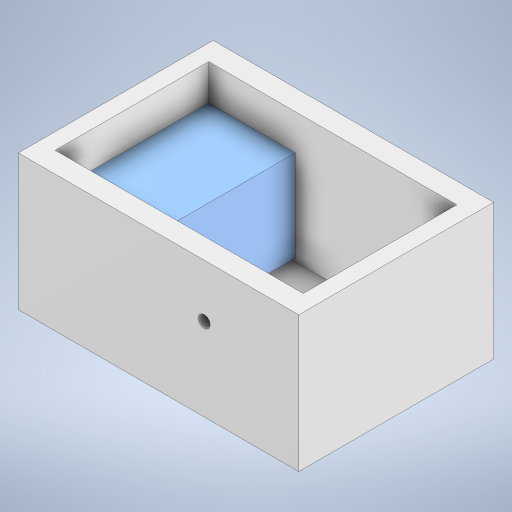
# Autodesk Inventor part: JunctionBox
Saved by Autodesk Inventor 2024.2 (Build 282272000, 272)
## iProperties
Created: 2024-01-15
Part Number: JunctionBox
Material: ABS Plastic
Document SubType Name: Modeling
Designer: airso
Density: 1.06 g/cm^3
Appearance: Smooth - White
Author: airso
Autodesk Inventor part; units mm, degrees
ref_plane "YZ Plane" through (0, 0, 0) normal (1, 0, 0) x (0, 1, 0)
ref_plane "XZ Plane" through (0, 0, 0) normal (0, 1, 0) x (-1, 0, 0)
ref_plane "XY Plane" through (0, 0, 0) normal (0, 0, 1) x (1, 0, 0)
sketch "Sketch1" plane through (0, 0, 0) normal (0, 1, 0) x (-1, 0, 0)
  line L0 (133.35, 82.55) -> (-133.35, 82.55)
  line L1 (-133.35, 82.55) -> (-133.35, -82.55)
  line L2 (-133.35, -82.55) -> (133.35, -82.55)
  line L3 (133.35, -82.55) -> (133.35, 82.55)
  line L4 (133.35, 82.55) -> (-133.35, -82.55) construction
  line L5 (-133.35, 82.55) -> (133.35, -82.55) construction
  line L6 (-150.8125, 104.775) -> (150.8125, 104.775)
  line L7 (150.8125, 104.775) -> (150.8125, -104.775)
  line L8 (150.8125, -104.775) -> (-150.8125, -104.775)
  line L9 (-150.8125, -104.775) -> (-150.8125, 104.775)
  line L10 (-150.8125, 104.775) -> (150.8125, -104.775) construction
  line L11 (150.8125, 104.775) -> (-150.8125, -104.775) construction
  point P0 (0, 0)
  dimension "d0" = 165.1
  dimension "d1" = 266.7
  dimension "d2" = 209.55
  dimension "d3" = 301.625
  constraints: 24 end point, 4 midpoint, 4 parallel, 2 horizontal, 2 perpendicular
  measures "d0" distance of L2.end L0.start
  measures "d1" distance of L1.end L2.end
  measures "d2" distance of L6.end L7.end
  measures "d3" distance of L6.start L6.end
extrude "Extrusion1" add sketch "Sketch1" along normal blind 146.05
sketch "Sketch2" plane through (0, 0, 0) normal (0, -1, 0) x (1, 0, 0)
  line L0 (133.35, 82.55) -> (-133.35, 82.55) projected
  line L1 (-133.35, -82.55) -> (133.35, -82.55) projected
  line L2 (-133.35, 82.55) -> (133.35, 82.55)
  line L3 (133.35, 82.55) -> (133.35, -82.55)
  line L4 (133.35, -82.55) -> (-133.35, -82.55)
  line L5 (-133.35, -82.55) -> (-133.35, 82.55)
  point P0 (0, 0)
  point P1 (133.35, 82.55)
  point P2 (-133.35, -82.55)
  constraints: 8 end point, 2 parallel, 1 horizontal, 1 perpendicular
extrude "Extrusion2" add sketch "Sketch2" against normal blind 3.175
sketch "Sketch3" plane through (0, 3.175, 0) normal (0, 1, 0) x (1, 0, 0)
  line L0 (-133.35, -82.55) -> (-133.35, 82.55) projected
  line L1 (-133.35, 82.55) -> (133.35, 82.55) projected
  line L2 (-133.35, -82.55) -> (133.35, -82.55)
  line L3 (133.35, -82.55) -> (133.35, 82.55)
  line L4 (133.35, 82.55) -> (-133.35, 82.55)
  line L5 (-133.35, 82.55) -> (-133.35, -82.55)
  line L6 (130.175, -79.375) -> (-130.175, -79.375)
  line L7 (-130.175, -79.375) -> (-130.175, 79.375)
  line L8 (-130.175, 79.375) -> (130.175, 79.375)
  line L9 (130.175, 79.375) -> (130.175, -79.375)
  point P0 (0, 0)
  dimension "d8" = 3.175
  constraints: 16 end point, 4 parallel, 2 perpendicular, 1 horizontal, 3 other
  measures "d8" distance between parallel lines of L2 L6
extrude "Extrusion3" add sketch "Sketch3" along normal blind 6.35 contours L6 L7 L8 L9
sketch "Sketch5" plane through (-133.35, 146.05, 82.55) normal (1, 0, 0) x (0, 0, -1)
  line L0 (0, -38.481) -> (165.1, -38.481)
  line L1 (165.1, -38.481) -> (14.224, -38.481)
  line L2 (14.224, -38.481) -> (14.224, -136.525)
  line L3 (14.224, -136.525) -> (165.1, -136.525)
  line L4 (165.1, -136.525) -> (165.1, -38.481)
  point P0 (82.55, -146.05)
  point P1 (165.1, -142.875)
  dimension "d15" = 98.044
  dimension "d16" = 150.876
  dimension "d19" = 6.35
  constraints: 10 end point, 2 parallel, 1 horizontal, 1 perpendicular
  measures "d15" distance of L1.end L2.end
  measures "d16" distance of L2.end L3.end
  measures "d19" distance from line of point (165.1, -142.875) L3
extrude "Extrusion5" add sketch "Sketch5" along normal blind 92.964
sketch "Sketch6" plane through (0, 9.525, 0) normal (0, 1, 0) x (1, 0, 0)
  line L0 (62.8142, 28.702) -> (-34.036, 28.702)
  line L1 (-34.036, 28.702) -> (-34.036, -79.375)
  line L2 (-34.036, -79.375) -> (62.8142, -79.375)
  line L3 (62.8142, -79.375) -> (62.8142, 28.702)
  line L4 (-130.175, -79.375) -> (130.175, -79.375) projected
  line L5 (-40.386, 82.55) -> (-40.386, -68.326) projected
  point P0 (0, 0)
  dimension "d20" = 108.077
  dimension "d21" = 96.8502
  dimension "d61" = 0
  dimension "d62" = 6.35
  constraints: 8 end point, 2 parallel, 1 horizontal, 1 perpendicular
  measures "d20" distance of L2.end L0.start
  measures "d21" distance of L1.end L2.end
  measures "d61" distance between parallel lines of L4 L2
  measures "d62" distance between parallel lines of L5 L1
extrude "Extrusion6" add sketch "Sketch6" along normal blind 3.175
sketch "Sketch8" plane through (0, 0, 0) normal (0, -1, 0) x (1, 0, 0)
  circle A0 centre (144.4625, 38.1) radius 3.4925
  line L0 (-150.8125, 104.775) -> (150.8125, 104.775) projected
  line L1 (150.8125, 104.775) -> (150.8125, -104.775) projected
  circle A1 centre (144.4625, -38.1) radius 3.4925
  line L2 (150.8125, -104.775) -> (-150.8125, -104.775) projected
  circle A2 centre (-144.4625, 38.1) radius 3.175
  circle A3 centre (-144.4625, -38.1) radius 3.4925
  line L3 (-150.8125, -104.775) -> (-150.8125, 104.775) projected
  line L4 (150.8125, 50.8) -> (-150.8125, 50.8)
  line L5 (150.8125, -50.8) -> (-150.8125, -50.8)
  point P0 (0, 0)
  dimension "d28" = 6.985
  dimension "d30" = 6.35
  dimension "d31" = 6.35
  dimension "d33" = 6.985
  dimension "d34" = 6.35
  dimension "d36" = 6.35
  dimension "d38" = 6.985
  dimension "d39" = 6.35
  dimension "d55" = 50.8
  dimension "d56" = 50.8
  dimension "d57" = 12.7
  dimension "d58" = 12.7
  dimension "d59" = 12.7
  dimension "d60" = 12.7
  constraints: 4 centre point, 4 end point, 4 point on line, 2 perpendicular
  measures "d28" diameter of A0
  measures "d30" distance from line of L1 A0.centre
  measures "d31" distance from line of L1 A1.centre
  measures "d33" diameter of A1
  measures "d34" distance from line of L3 A2.centre
  measures "d36" distance from line of L3 A3.centre
  measures "d38" diameter of A3
  measures "d39" diameter of A2
  measures "d55" distance from line of L4 point (0, 0)
  measures "d56" distance from line of L5 point (0, 0)
  measures "d57" distance from line of L4 A0.centre
  measures "d58" distance from line of L5 A1.centre
  measures "d59" distance from line of L4 A2.centre
  measures "d60" distance from line of L5 A3.centre
extrude "Extrusion8" cut sketch "Sketch8" against normal blind 6.35 contours A0 | A1 | A2 | A3
sketch "Sketch11" plane through (0, 12.7, 0) normal (0, 1, 0) x (1, 0, 0)
  circle A0 centre (56.2991, 19.7485) radius 1.7018
  circle A1 centre (56.2991, -70.4215) radius 1.7018
  circle A2 centre (-27.5209, 19.7485) radius 1.7018
  circle A3 centre (-27.5209, -70.4215) radius 1.7018
  line L0 (62.8142, 28.702) -> (-34.036, 28.702) projected
  line L1 (-34.036, -79.375) -> (62.8142, -79.375) projected
  line L2 (62.8142, -79.375) -> (62.8142, 28.702) projected
  line L3 (-34.036, 28.702) -> (-34.036, -79.375) projected
  point P0 (0, 0)
  dimension "d82" = 3.4036
  dimension "d83" = 83.82
  dimension "d85" = 83.82
  dimension "d87" = 6.5151
  dimension "d88" = 6.5151
  dimension "d89" = 90.17
  dimension "d90" = 8.9535
  dimension "d91" = 3.4036
  dimension "d92" = 3.4036
  dimension "d93" = 3.4036
  constraints: 4 centre point
  measures "d82" diameter of A0
  measures "d83" distance of A2.centre A0.centre
  measures "d85" distance of A3.centre A1.centre
  measures "d87" distance from line of L2 A0.centre
  measures "d88" distance from line of L2 A1.centre
  measures "d89" distance of A0.centre A1.centre
  measures "d90" distance from line of L1 A1.centre
  measures "d91" diameter of A2
  measures "d92" diameter of A3
  measures "d93" diameter of A1
extrude "Extrusion11" cut sketch "Sketch11" against normal up to surface (3.175 mm away) contours A0 | A1 | A2 | A3
sketch "Sketch12" plane through (-150.8125, 0, 104.775) normal (0, 0, 1) x (1, 0, 0)
  circle A0 centre (200.025, 89.154) radius 6.35
  line L0 (301.625, 0) -> (301.625, 146.05) projected
  line L1 (0, 146.05) -> (301.625, 146.05) projected
  point P0 (150.8125, 0)
  dimension "d77" = 12.7
  dimension "d78" = 101.6
  dimension "d79" = 56.896
  constraints: 1 centre point
  measures "d77" diameter of A0
  measures "d78" distance from line of L0 A0.centre
  measures "d79" distance from line of L1 A0.centre
extrude "Extrusion12" cut sketch "Sketch12" against normal up to surface (22.225 mm away)
body "Solid1"
